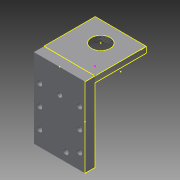
# Autodesk Inventor part: DetectionAdapter
Saved by Autodesk Inventor 2013 (Build 170138000, 138)
## iProperties
Created: 2014-06-27
Part Number: DetectionAdapter
Material: Generic
Document SubType Name: Modeling
Designer: 120pa
Density: 1 g/cm^3
Author: 120pa
Autodesk Inventor part; units mm, degrees
ref_plane "YZ Plane" through (0, 0, 0) normal (1, 0, 0) x (0, 1, 0)
ref_plane "XZ Plane" through (0, 0, 0) normal (0, 1, 0) x (-1, 0, 0)
ref_plane "XY Plane" through (0, 0, 0) normal (0, 0, 1) x (1, 0, 0)
sketch "Sketch1" plane through (0, 0, 0) normal (0, 1, 0) x (-1, 0, 0)
  line L0 (-32.512, -44.196) -> (32.512, -44.196)
  line L1 (32.512, -44.196) -> (32.512, 44.196)
  line L2 (32.512, 44.196) -> (-32.512, 44.196)
  line L3 (-32.512, 44.196) -> (-32.512, -44.196)
  line L4 (-32.512, -44.196) -> (32.512, 44.196) construction
  line L5 (32.512, -44.196) -> (-32.512, 44.196) construction
  point P0 (0, 0)
  point P1 (0, 0)
  dimension "d0" = 65.024
  dimension "d1" = 88.392
  constraints: 12 end point, 2 midpoint
  measures "d0" distance of L2.end L1.end
  measures "d1" distance of L1.end L0.end
extrude "Extrusion1" add sketch "Sketch1" along normal blind 12.7
hole "Hole1" at (-25.4, 12.7, -37.084) direction (0, -1, 0) diameter 6.7564 end through all clearance for "Flat Head Machine Screw (82)" size "1/4" standard "Ansi Unified Screw Threads"
hole "Hole3" at (25.4, 12.7, -37.084) direction (0, -1, 0) diameter 6.7564 end through all clearance for "Flat Head Machine Screw (82)" size "1/4" standard "Ansi Unified Screw Threads"
hole "Hole4" at (25.4, 12.7, -11.684) direction (0, -1, 0) diameter 6.7564 end through all clearance for "Flat Head Machine Screw (82)" size "1/4" standard "Ansi Unified Screw Threads"
hole "Hole5" at (25.4, 12.7, 13.716) direction (0, -1, 0) diameter 6.7564 end through all clearance for "Flat Head Machine Screw (82)" size "1/4" standard "Ansi Unified Screw Threads"
hole "Hole6" at (0, 12.7, 13.716) direction (0, -1, 0) diameter 6.7564 end through all clearance for "Flat Head Machine Screw (82)" size "1/4" standard "Ansi Unified Screw Threads"
hole "Hole7" at (-25.4, 12.7, 13.716) direction (0, -1, 0) diameter 6.7564 end through all clearance for "Flat Head Machine Screw (82)" size "1/4" standard "Ansi Unified Screw Threads"
hole "Hole8" at (-25.4, 12.7, -11.684) direction (0, -1, 0) diameter 6.7564 end through all clearance for "Flat Head Machine Screw (82)" size "1/4" standard "Ansi Unified Screw Threads"
sketch "Sketch2" plane through (0, 12.7, 0) normal (0, 1, 0) x (1, 0, 0)
  line L0 (-32.512, -44.5719) -> (32.512, -44.196)
  line L1 (32.512, -44.196) -> (25.4, -36.614)
  line L2 (25.4, -36.614) -> (-25.4, -36.614)
  line L3 (-25.4, -36.614) -> (-32.512, -44.5719)
  line L4 (-32.512, -44.5719) -> (25.4, -36.614) construction
  line L5 (32.512, -44.196) -> (-25.4, -36.614) construction
  point P0 (0, 0)
  point P1 (0.6144, -40.0199)
  constraints: 12 end point, 2 point on line
extrude "Extrusion2" add sketch "Sketch2" along normal blind 65.278
hole "Hole9" at (-0.0005, 52.578, 44.384) direction (-0.0057808, 0, -0.9999833) diameter 23.9268 end through all
sketch "Sketch3" plane through (32.512, 0, -44.196) normal (0, 0, -1) x (-1, 0, 0)
  line L0 (0, 12.7) -> (65.024, 12.7)
  line L1 (65.024, 12.7) -> (65.024, 0)
  line L2 (65.024, 0) -> (0, 0)
  line L3 (0, 0) -> (0, 12.7)
  line L4 (0, 12.7) -> (65.024, 0) construction
  line L5 (65.024, 12.7) -> (0, 0) construction
  point P0 (32.512, 0)
  point P1 (32.512, 6.35)
  constraints: 12 end point, 2 midpoint
extrude "Extrusion3" add sketch "Sketch3" along normal blind 12.7
hole "Hole10" at (8.0772, 0, -45.166) direction (0, 1, 0) diameter 4.318 end through all counterbore diameter 7.112 counterbore depth 5.588
hole "Hole13" at (12.7, 12.7, 0.635) direction (0, -1, 0) diameter 4.9784 depth 7.62 tip angle 118 thread size "1/4-20 UNC" class "2B" standard "ANSI Unified Screw Threads"
hole "Hole14" at (-12.7, 12.7, 0.635) direction (0, -1, 0) diameter 4.9784 depth 7.62 tip angle 118 thread size "1/4-20 UNC" class "2B" standard "ANSI Unified Screw Threads"
sketch "Sketch4" plane through (32.512, 12.7, 36.614) normal (1, 0, 0) x (0, 0, -1)
  line L0 (-7.582, -12.7) -> (93.51, -12.7) projected
  line L1 (93.51, 0) -> (93.51, -12.7) projected
  line L2 (0, 0) -> (93.51, 0) projected
  line L3 (0, 0) -> (0, 65.278) projected
  line L4 (-7.582, 65.278) -> (0, 65.278) projected
  line L5 (-7.582, 0) -> (-7.582, 65.278) projected
  line L6 (-18.542, 0) -> (-18.1661, 0) projected
  line L7 (-7.582, -12.7) -> (-7.582, 0) projected
  point P0 (36.614, -12.7)
  constraints: 2 other
sketch "Sketch5" plane through (32.512, 12.7, 36.614) normal (1, 0, 0) x (0, 0, -1)
  line L0 (-7.582, -12.7) -> (93.51, -12.7) projected
  line L1 (93.51, 0) -> (93.51, -12.7) projected
  line L2 (0, 0) -> (93.51, 0) projected
  line L3 (0, 0) -> (0, 65.278) projected
  line L4 (-7.582, 65.278) -> (0, 65.278) projected
  line L5 (-7.582, 0) -> (-7.582, 65.278) projected
  line L6 (-18.542, 0) -> (-18.1661, 0) projected
  line L7 (-7.582, -12.7) -> (-7.582, 0) projected
  point P0 (36.614, -12.7)
  constraints: 2 other
sketch "Sketch6" plane through (0, 77.978, 0) normal (0, 1, 0) x (1, 0, 0)
  line L0 (-32.512, -44.5719) -> (32.512, -44.196) projected
  line L1 (32.512, -44.196) -> (25.4, -36.614) projected
  line L2 (25.4, -36.614) -> (-25.4, -36.614) construction
  line L3 (-25.4, -36.614) -> (-32.512, -44.5719) projected
  point P0 (0, 0)
sketch "Sketch7" plane through (32.512, 12.7, 36.614) normal (1, 0, 0) x (0, 0, -1)
  line L0 (-7.582, -12.7) -> (93.51, -12.7) projected
  line L1 (93.51, 0) -> (93.51, -12.7) projected
  line L2 (0, 0) -> (93.51, 0) projected
  line L3 (0, 0) -> (0, 65.278) projected
  line L4 (-7.582, 65.278) -> (0, 65.278) projected
  line L5 (-7.582, 0) -> (-7.582, 65.278) construction
  line L6 (-18.542, 0) -> (-18.1661, 0) projected
  line L7 (-7.582, -12.7) -> (-7.582, 0) projected
  point P0 (36.614, -12.7)
  constraints: 2 other
sketch "Sketch8" plane through (-32.512, 12.7, 44.5719) normal (0.0057808, 0, 0.9999833) x (0.9999833, 0, -0.0057808)
  circle A0 centre (32.512, 39.878) radius 11.9634 projected
  line L0 (0, 0) -> (65.0251, 0) projected
  line L1 (65.0251, 0) -> (65.0251, 65.278) projected
  line L2 (0, 65.278) -> (65.0251, 65.278) projected
  line L3 (0, 0) -> (0, 65.278) projected
  point P0 (65.024, 0)
  point P1 (32.7691, -12.7)
  constraints: 1 other
hole "Hole16" at (12.7, 12.7, -24.765) direction (0, -1, 0) diameter 4.9784 depth 7.62 tip angle 118 thread size "1/4-20 UNC" class "2B" standard "ANSI Unified Screw Threads"
hole "Hole17" at (-12.7, 12.7, -24.765) direction (0, -1, 0) diameter 4.9784 depth 7.62 tip angle 118 thread size "1/4-20 UNC" class "2B" standard "ANSI Unified Screw Threads"
body "Solid1"
